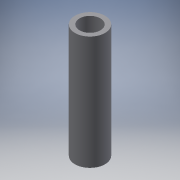
# Autodesk Inventor part: arms_link_001
Saved by Autodesk Inventor 2016 SP1 (Build 200210100, 210)
## iProperties
Created: 2016-06-22
Part Number: arms_link_001
Material: Generic
Document SubType Name: Modeling
Designer: asvsf
Density: 1 g/cm^3
Appearance: Default
Author: asvsf
Autodesk Inventor part; units mm, degrees
ref_plane "YZ Plane" through (0, 0, 0) normal (1, 0, 0) x (0, 1, 0)
ref_plane "XZ Plane" through (0, 0, 0) normal (0, 1, 0) x (-1, 0, 0)
ref_plane "XY Plane" through (0, 0, 0) normal (0, 0, 1) x (1, 0, 0)
sketch "Sketch1" plane through (0, 0, 0) normal (0, 1, 0) x (-1, 0, 0)
  circle A0 centre (0, 0) radius 13
  circle A1 centre (0, 0) radius 9
  dimension "d0" = 26
  dimension "d3" = 18
  constraints: 2 centre point, 2 coincident
  measures "d0" diameter of A0
  measures "d3" diameter of A1
extrude "Extrusion1" add sketch "Sketch1" along normal mid plane 98.4
body "Solid1"
